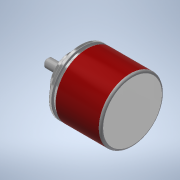
# Autodesk Inventor part: opkon_encoder
Saved by Autodesk Inventor 2021 (Build 250183000, 183)
## iProperties
Created: 2022-06-02
Part Number: opkon_encoder
Material: Stahl
Document SubType Name: Modeling
Designer: 10154704
Density: 7.85 g/cm^3
Appearance: Stahl
Author: 10154704
Autodesk Inventor part; units mm, degrees
ref_plane "YZ Plane" through (0, 0, 0) normal (1, 0, 0) x (0, 1, 0)
ref_plane "XZ Plane" through (0, 0, 0) normal (0, 1, 0) x (-1, 0, 0)
ref_plane "XY Plane" through (0, 0, 0) normal (0, 0, 1) x (1, 0, 0)
sketch "Skizze1" plane through (0, 0, 0) normal (0, 0, 1) x (1, 0, 0)
  line L0 (0, 0) -> (0, 4)
  line L1 (0, 4) -> (20, 4)
  line L2 (20, 4) -> (20, 18)
  line L3 (20, 18) -> (30, 18)
  line L4 (30, 18) -> (30, 29)
  line L5 (30, 29) -> (33, 29)
  line L6 (33, 29) -> (33, 27)
  line L7 (33, 27) -> (36, 27)
  line L8 (36, 27) -> (36, 29)
  line L9 (36, 29) -> (78, 29)
  line L10 (78, 29) -> (78, 0)
  line L11 (78, 0) -> (0, 0)
  dimension "d0" = 8
  dimension "d1" = 36
  dimension "d2" = 54
  dimension "d3" = 58
  dimension "d4" = 20
  dimension "d5" = 10
  dimension "d6" = 3
  dimension "d7" = 3
  dimension "d8" = 42
  constraints: 24 end point, 10 perpendicular, 2 point on line, 1 vertical
  measures "d0" diameter of L1 L11
  measures "d1" diameter of L3 L11
  measures "d2" diameter of L7 L11
  measures "d3" diameter of L9 L11
  measures "d4" distance between parallel lines of L2 L0
  measures "d5" distance between parallel lines of L2 L4
  measures "d6" distance between parallel lines of L4 L6
  measures "d7" distance between parallel lines of L8 L6
  measures "d8" distance between parallel lines of L10 L8
revolve "Umdrehung1" add sketch "Skizze1" angle 360 about axis through (78, 0, 0) along (-1, 0, 0)
fillet "Rundung1" radius 2 1 edges at (78, -29, 0)
fillet "Rundung1" radius 0.5 4 edges at (20, -18, 0) (30, -29, 0) (36, -29, 0) (33, -29, 0)
chamfer "Fase1" distance 1 angle 45 1 edges at (0, -4, 0)
sketch "Skizze3" plane through (30, 0, 0) normal (-1, 0, 0) x (0, 0, 1)
  circle A0 centre (0, 0) radius 4 projected
  line L0 (0, 0) -> (24, 0)
  dimension "d18" = 24
  constraints: 2 end point, 1 coincident, 1 horizontal
  measures "d18" distance of point (0, 0) point (24, 0)
hole "Bohrung1" at (30, 0, 24) direction (1, 0, 0) diameter 2.459 depth 8.8 tip angle 118 thread size "M3x0.5" class "6H" standard "ISO Metric profile"
pattern_circular "Runde Anordnung1" count 3 over 360 about axis through (10, 0, 0) along (1, 0, 0) of "Bohrung1"
sketch "Skizze4" plane through (0, 0, 0) normal (0, 1, 0) x (-1, 0, 0)
  line L0 (-76, 29) -> (-76, -29) projected
  line L1 (-36.5, -29) -> (-36.5, 29) projected
  line L2 (-66.1876, -34.3335) -> (-63.5778, -34.3335)
  line L3 (-63.5778, -34.3335) -> (-63.5778, -30.1897)
  line L4 (-63.5778, -30.1897) -> (-66.1876, -30.1897)
  line L5 (-66.1876, -30.1897) -> (-66.1876, -34.3335)
  line L6 (-66.1876, -30.1897) -> (-59.995, -30.1897)
  line L7 (-59.995, -30.1897) -> (-59.995, -26.9412)
  line L8 (-59.995, -26.9412) -> (-66.1876, -26.9412)
  line L9 (-66.1876, -26.9412) -> (-66.1876, -30.1897)
  point P0 (0, 0)
  constraints: 16 end point, 4 parallel, 2 horizontal, 2 perpendicular
revolve "Umdrehung2" add sketch "Skizze4" angle 360 about axis through (66.1876, 0, -30.1897) along (0, 0, -1)
fillet "Rundung2" radius 0.5 2 edges at (72.3802, 0, -30.1897) (68.7974, 0, -30.1897)
sketch "Sketch5" plane through (0, 0, 0) normal (-1, 0, 0) x (0, 0, 1)
  circle A0 centre (0, 0) radius 4 projected
  circle A1 centre (0, 0) radius 4 projected
  line L0 (-3, 2.6458) -> (-3, -2.6458)
  arc A2 (-3, 2.6458) -> (-3, -2.6458) centre (0, 0) ccw
  dimension "d37" = 3
  constraints: 4 point on circle, 2 end point, 1 centre point, 1 concentric, 1 vertical
  measures "d37" distance from line of point (0, 0) L0
extrude "Extrusion2" cut sketch "Sketch5" against normal blind 11 contours L0 A0 picked at (-3.1815, -0.6179)
